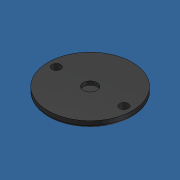
# Autodesk Inventor part: ANTI-SKID PAD 100mm WITH ATTACHMENT BORES
Saved by Autodesk Inventor 2016 (Build 200138000, 138)
## iProperties
Created: 2007-03-28
Part Number: ANTI-SKID PAD 100mm WITH ATTACHMENT BORES
Material: Rubber
Document SubType Name: Modeling
Designer: Andy Moles
Density: 0.93 g/cm^3
Appearance: Rubber - Black - Version 1.1
Author: Andy Moles
Autodesk Inventor part; units mm, degrees
ref_plane "YZ Plane" through (0, 0, 0) normal (1, 0, 0) x (0, 1, 0)
ref_plane "XZ Plane" through (0, 0, 0) normal (0, 1, 0) x (-1, 0, 0)
ref_plane "XY Plane" through (0, 0, 0) normal (0, 0, 1) x (1, 0, 0)
sketch "Sketch1" plane through (0, 0, 0) normal (0, 0, 1) x (1, 0, 0)
  circle A0 centre (0, 0) radius 46
  circle A1 centre (-37, 0) radius 4.75
  circle A2 centre (37, 0) radius 4.75
  dimension "d0" = 92
  dimension "d7" = 9.5
  dimension "d8" = 9.5
  dimension "d9" = 74
  dimension "d10" = 37
  constraints: 3 centre point, 2 horizontal alignment, 1 coincident
  measures "d0" diameter of A0
  measures "d7" diameter of A1
  measures "d8" diameter of A2
  measures "d9" distance of A2.centre A1.centre
  measures "d10" distance of point (0, 0) A1.centre
extrude "Extrusion1" add sketch "Sketch1" along normal blind 7
sketch "Sketch2" plane through (0, 0, 7) normal (0, 0, 1) x (1, 0, 0)
  circle A0 centre (0, 0) radius 46 projected
  circle A1 centre (0, 0) radius 7.5
  dimension "d3" = 15
  constraints: 1 centre point, 1 coincident
  measures "d3" diameter of A1
extrude "Extrusion2" cut sketch "Sketch2" against normal blind 4 contours A1
fillet "Fillet1" radius 2.5 1 edges at (-46, 0, 0)
equation "\"d10\" = 0.5 * d9"
body "Solid1"
